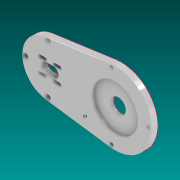
# Autodesk Inventor part: base bovenkant
Saved by Autodesk Inventor 2020.2 (Build 242310000, 310)
## iProperties
Created: 2020-05-15
Part Number: base bovenkant
Material: Aluminum 6061
Document SubType Name: Modeling
Designer: Svend
Density: 2.7 g/cm^3
Appearance: Aluminum - Polished
Author: Svend
Autodesk Inventor part; units mm, degrees
ref_plane "YZ Plane" through (0, 0, 0) normal (1, 0, 0) x (0, 1, 0)
ref_plane "XZ Plane" through (0, 0, 0) normal (0, 1, 0) x (-1, 0, 0)
ref_plane "XY Plane" through (0, 0, 0) normal (0, 0, 1) x (1, 0, 0)
sketch "Sketch1" plane through (0, 0, 0) normal (0, 0, 1) x (1, 0, 0)
  circle A0 centre (-11.3135, -11.3135) radius 2
  circle A1 centre (-11.3135, 11.3135) radius 2
  circle A2 centre (11.3135, 11.3135) radius 2
  circle A3 centre (11.3135, -11.3135) radius 2
  circle A4 centre (-15.3135, 11.3135) radius 2
  circle A5 centre (-7.3135, 11.3135) radius 2
  circle A6 centre (7.3135, 11.3135) radius 2
  circle A7 centre (15.3135, 11.3135) radius 2
  circle A8 centre (15.3135, -11.3135) radius 2
  circle A9 centre (7.3135, -11.3135) radius 2
  circle A10 centre (-7.3135, -11.3135) radius 2
  circle A11 centre (-15.3135, -11.3135) radius 2
  line L0 (-15.3135, 13.3135) -> (-7.3135, 13.3135)
  line L1 (-7.3135, 9.3135) -> (-15.3135, 9.3135)
  line L2 (-15.3135, -9.3135) -> (-7.3135, -9.3135)
  line L3 (-7.3135, -13.3135) -> (-15.3135, -13.3135)
  line L4 (7.3135, -9.3135) -> (15.3135, -9.3135)
  line L5 (15.3135, -13.3135) -> (7.3135, -13.3135)
  line L6 (15.3135, 9.3135) -> (7.3135, 9.3135)
  line L7 (15.3135, 13.3135) -> (7.3135, 13.3135)
  circle A12 centre (0, 0) radius 8.25
  circle A13 centre (5, 0) radius 8.25
  circle A14 centre (-5, 0) radius 8.25
  line L8 (-5, 8.25) -> (5, 8.25)
  line L9 (5, -8.25) -> (-5, -8.25)
  circle A15 centre (0, 0) radius 42.5
  circle A16 centre (100.143, 0) radius 56.4372
  line L10 (-5.9149, 42.0864) -> (92.2885, 55.888)
  line L11 (-5.9149, -42.0864) -> (92.2885, -55.888)
  line L12 (-13.25, 0) -> (13.25, 0)
  circle A17 centre (100.143, 0) radius 11.5
  arc A18 (-5.9149, 42.0864) -> (-5.9149, -42.0864) centre (0, 0) ccw
  arc A19 (92.2885, -55.888) -> (92.2885, 55.888) centre (100.143, 0) ccw
  line L13 (-42.5, 0) -> (156.5802, 0)
  line L14 (92.2885, 55.888) -> (-5.9149, 42.0864)
  line L15 (-5.9149, -42.0864) -> (92.2885, -55.888)
  line L16 (-3.1314, 22.281) -> (95.0719, 36.0826)
  arc A20 (95.0719, -36.0826) -> (95.0719, 36.0826) centre (100.143, 0) ccw
  line L17 (95.0719, -36.0826) -> (-3.1314, -22.281)
  arc A21 (-3.1314, 22.281) -> (-3.1314, -22.281) centre (0, 0) ccw
  point P0 (151.5802, 0)
  point P1 (95.0719, 51.23)
  point P2 (95.0719, -51.23)
  point P3 (-37.5, 0)
  point P4 (-3.1314, 37.4284)
  point P5 (-3.1314, -37.4284)
  dimension "d0" = 4
  dimension "d1" = 22.627
  dimension "d2" = 22.627
  dimension "d3" = 11.3135
  dimension "d4" = 11.3135
  dimension "d5" = 4
  dimension "d6" = 4
  dimension "d7" = 4
  dimension "d8" = 4
  dimension "d9" = 4
  dimension "d10" = 4
  dimension "d11" = 4
  dimension "d12" = 4
  dimension "d15" = 16.5
  dimension "d16" = 5
  dimension "d17" = 5
  dimension "d18" = 85
  dimension "d19" = 8
  dimension "d20" = 100.143
  dimension "d21" = 23
  dimension "d24" = 85
  dimension "d25" = 100.143
  dimension "d26" = 8
  dimension "d27" = 20
  dimension "d28" = 15
  dimension "d29" = 5
  dimension "d30" = 15
  dimension "d31" = 15
  dimension "d32" = 15
  dimension "d33" = 5
  constraints: 36 end point, 36 point on circle, 22 centre point, 15 horizontal alignment, 14 tangent, 13 equal radius, 11 point on line, 6 vertical alignment, 4 coincident, 4 parallel, 3 horizontal, 1 midpoint, 3 other
  measures "d0" diameter of A0
  measures "d1" distance of A1.centre A2.centre
  measures "d2" distance of A3.centre A2.centre
  measures "d3" horizontal distance of point (0, 0) A1.centre
  measures "d4" horizontal distance of point (0, 0) A1.centre
  measures "d5" distance of A2.centre A6.centre
  measures "d6" distance of A7.centre A2.centre
  measures "d7" distance of A3.centre A8.centre
  measures "d8" distance of A9.centre A3.centre
  measures "d9" distance of A0.centre A10.centre
  measures "d10" distance of A11.centre A0.centre
  measures "d11" distance of A1.centre A4.centre
  measures "d12" distance of A5.centre A1.centre
  measures "d15" diameter of A12
  measures "d16" distance of A14.centre A12.centre
  measures "d17" distance of A12.centre A13.centre
  measures "d18" diameter of A15
  measures "d19" angle of L12 L10
  measures "d20" distance of A16.centre point (0, 0)
  measures "d21" diameter of A17
  measures "d24" diameter of A18
  measures "d25" distance of A18.centre A19.centre
  measures "d26" angle of L13 L14
  measures "d27" distance between parallel lines of L14 L16
  measures "d28" distance from line of point (-3.131, -37.428) L17
  measures "d29" distance of L13.end point (151.58, 0)
  measures "d30" distance from line of L16 point (95.072, 51.23)
  measures "d31" distance from line of L16 point (-3.131, 37.428)
  measures "d32" distance from line of point (95.072, -51.23) L17
  measures "d33" distance of L13.start point (-37.5, 0)
extrude "Extrusion1" add sketch "Sketch1" along normal blind 10 contours L13 A15 L17 A21 A14 L9 A13 | A13 L8 A14 L13 A21 L16 A15 | L13 A16 L17 A15 | A15 L16 A16 L13 | L16 A21 L13 A15 | A15 L10 A16 L16 | L17 A16 L11 A15 | A15 L13 A21 L17 | L13 A17 A20 L17 A16 | A16 L16 A20 L13 A17 | A16 L13 A20 L16 | L17 A20 L13 A16
hole "Hole1" at (-3.1314, -37.4284, 0) at (95.0719, -51.23, 0) at (151.5802, 0, 0) at (95.0719, 51.23, 0) at (-3.1314, 37.4284, 0) at (-37.5, 0, 0) direction (0, 0, 1) diameter 5.2 depth 10 tip angle 118
chamfer "Chamfer1" distance 0.5 angle 45 28 edges at (-42.5, 0, 10) (43.1868, -48.9872, 10) (156.5802, 0, 10) (43.1868, 48.9872, 10) (-5.3135, 11.3135, 10) (-11.3135, 9.3135, 10) (-17.3135, 11.3135, 10) (-11.3135, 13.3135, 10) (-13.25, 0, 10) (0, 8.25, 10) (13.25, 0, 10) (0, -8.25, 10) (-11.3135, -9.3135, 10) (-5.3135, -11.3135, 10) (-11.3135, -13.3135, 10) (-17.3135, -11.3135, 10) (5.3135, 11.3135, 10) (11.3135, 13.3135, 10) (17.3135, 11.3135, 10) (11.3135, 9.3135, 10) (17.3135, -11.3135, 10) (11.3135, -13.3135, 10) (5.3135, -11.3135, 10) (11.3135, -9.3135, 10) (88.643, 0, 10) (95.0719, -53.83, 10) (151.5802, -2.6, 10) (95.0719, 48.63, 10)
chamfer "Chamfer3" distance 2 angle 45 3 edges at (-3.1314, 34.8284, 10) (-37.5, -2.6, 10) (-3.1314, -40.0284, 10)
sketch "Sketch2" plane through (0, 0, 10) normal (0, 0, 1) x (1, 0, 0)
  arc A0 (-41.9879, -1.0095) -> (-41.9879, 1.0095) centre (-37.5, 0) ccw projected
  circle A1 centre (95.0719, 51.23) radius 3.1 projected
  circle A2 centre (95.0719, -51.23) radius 3.1 projected
  arc A3 (15.3135, -13.8135) -> (15.3135, -8.8135) centre (15.3135, -11.3135) ccw projected
  line L0 (7.3135, -13.8135) -> (15.3135, -13.8135) projected
  arc A4 (7.3135, -8.8135) -> (7.3135, -13.8135) centre (7.3135, -11.3135) ccw projected
  line L1 (15.3135, -8.8135) -> (7.3135, -8.8135) projected
  line L2 (-7.3135, -8.8135) -> (-15.3135, -8.8135) projected
  arc A5 (-7.3135, -13.8135) -> (-7.3135, -8.8135) centre (-7.3135, -11.3135) ccw projected
  line L3 (-15.3135, -13.8135) -> (-7.3135, -13.8135) projected
  arc A6 (-15.3135, -8.8135) -> (-15.3135, -13.8135) centre (-15.3135, -11.3135) ccw projected
  arc A7 (-7.3135, 8.8135) -> (-7.3135, 13.8135) centre (-7.3135, 11.3135) ccw projected
  line L4 (-15.3135, 8.8135) -> (-7.3135, 8.8135) projected
  arc A8 (-15.3135, 13.8135) -> (-15.3135, 8.8135) centre (-15.3135, 11.3135) ccw projected
  line L5 (-7.3135, 13.8135) -> (-15.3135, 13.8135) projected
  arc A9 (-41.9879, -1.0095) -> (-5.8453, -41.5913) centre (0, 0) ccw projected
  line L6 (92.358, -55.3928) -> (-2.813, -42.0174) projected
  arc A10 (92.358, -55.3928) -> (92.358, 55.3928) centre (100.143, 0) ccw projected
  line L7 (-5.8453, 41.5913) -> (-4.7023, 41.7519) projected
  arc A11 (-5, 8.75) -> (-5, -8.75) centre (-5, 0) ccw projected
  line L8 (5, 8.75) -> (-5, 8.75) projected
  arc A12 (5, -8.75) -> (5, 8.75) centre (5, 0) ccw projected
  line L9 (-5, -8.75) -> (5, -8.75) projected
  arc A13 (7.3135, 13.8135) -> (7.3135, 8.8135) centre (7.3135, 11.3135) ccw projected
  line L10 (15.3135, 13.8135) -> (7.3135, 13.8135) projected
  arc A14 (15.3135, 8.8135) -> (15.3135, 13.8135) centre (15.3135, 11.3135) ccw projected
  line L11 (7.3135, 8.8135) -> (15.3135, 8.8135) projected
  circle A15 centre (100.143, 0) radius 12 projected
  circle A16 centre (151.5802, 0) radius 3.1 projected
  arc A17 (-4.7023, 41.7519) -> (-2.813, 42.0174) centre (-3.1314, 37.4284) ccw projected
  arc A18 (-2.813, -42.0174) -> (-4.7023, -41.7519) centre (-3.1314, -37.4284) ccw projected
  circle A19 centre (100.143, 0) radius 35.05
  line L12 (-2.813, 42.0174) -> (92.358, 55.3928) projected
  arc A20 (-5.8453, 41.5913) -> (-41.9879, 1.0095) centre (0, 0) ccw projected
  line L13 (-4.7023, -41.7519) -> (-5.8453, -41.5913) projected
  dimension "d50" = 70.1
  constraints: 1 centre point, 1 coincident
  measures "d50" diameter of A19
extrude "Extrusion2" cut sketch "Sketch2" against normal blind 5 contours A15 | A19
chamfer "Chamfer4" distance 1 angle 45 2 edges at (65.093, 0, 10) (88.643, 0, 5)
sketch "Sketch3" plane through (0, 0, 0) normal (0, 0, -1) x (-1, 0, 0)
  circle A0 centre (3.1314, 37.4284) radius 2.6 projected
  circle A1 centre (-151.5802, 0) radius 2.6 projected
  circle A2 centre (3.1314, -37.4284) radius 2.6 projected
  circle A3 centre (-95.0719, -51.23) radius 2.6 projected
  circle A4 centre (-95.0719, 51.23) radius 2.6 projected
  circle A5 centre (37.5, 0) radius 2.6 projected
  line L0 (5.9149, -42.0864) -> (-92.2885, -55.888) projected
  arc A6 (5.9149, -42.0864) -> (5.9149, 42.0864) centre (0, 0) ccw projected
  line L1 (-92.2885, 55.888) -> (5.9149, 42.0864) projected
  arc A7 (-92.2885, 55.888) -> (-92.2885, -55.888) centre (-100.143, 0) ccw projected
  circle A8 centre (-100.143, 0) radius 11.5 projected
  line L2 (7.3135, 9.3135) -> (15.3135, 9.3135) projected
  arc A9 (7.3135, 13.3135) -> (7.3135, 9.3135) centre (7.3135, 11.3135) ccw projected
  line L3 (15.3135, 13.3135) -> (7.3135, 13.3135) projected
  arc A10 (15.3135, 9.3135) -> (15.3135, 13.3135) centre (15.3135, 11.3135) ccw projected
  line L4 (7.3135, -13.3135) -> (15.3135, -13.3135) projected
  arc A11 (7.3135, -9.3135) -> (7.3135, -13.3135) centre (7.3135, -11.3135) ccw projected
  line L5 (15.3135, -9.3135) -> (7.3135, -9.3135) projected
  arc A12 (15.3135, -13.3135) -> (15.3135, -9.3135) centre (15.3135, -11.3135) ccw projected
  line L6 (-15.3135, -13.3135) -> (-7.3135, -13.3135) projected
  arc A13 (-15.3135, -9.3135) -> (-15.3135, -13.3135) centre (-15.3135, -11.3135) ccw projected
  line L7 (-7.3135, -9.3135) -> (-15.3135, -9.3135) projected
  arc A14 (-7.3135, -13.3135) -> (-7.3135, -9.3135) centre (-7.3135, -11.3135) ccw projected
  line L8 (-7.3135, 13.3135) -> (-15.3135, 13.3135) projected
  arc A15 (-7.3135, 9.3135) -> (-7.3135, 13.3135) centre (-7.3135, 11.3135) ccw projected
  line L9 (-15.3135, 9.3135) -> (-7.3135, 9.3135) projected
  arc A16 (-15.3135, 13.3135) -> (-15.3135, 9.3135) centre (-15.3135, 11.3135) ccw projected
  line L10 (-5, -8.25) -> (5, -8.25) projected
  arc A17 (-5, 8.25) -> (-5, -8.25) centre (-5, 0) ccw projected
  line L11 (5, 8.25) -> (-5, 8.25) projected
  arc A18 (5, -8.25) -> (5, 8.25) centre (5, 0) ccw projected
  line L12 (-93.6802, -45.9853) -> (4.5231, -32.1837)
  arc A19 (4.5231, -32.1837) -> (4.5231, 32.1837) centre (0, 0) ccw
  line L13 (4.5231, 32.1837) -> (-93.6802, 45.9853)
  arc A20 (-93.6802, 45.9853) -> (-93.6802, -45.9853) centre (-100.143, 0) ccw
  dimension "d56" = 10
  constraints: 4 end point, 4 point on circle, 2 centre point, 3 other
  measures "d56" distance between parallel lines of L0 L12
equation "\"d2\" = d1"
equation "\"d3\" = 0.5 * d2"
equation "\"d4\" = 0.5 * d1"
equation "\"d5\" = d0"
equation "\"d6\" = d5"
equation "\"d7\" = d6"
equation "\"d8\" = d7"
equation "\"d9\" = d5"
equation "\"d10\" = d9"
equation "\"d11\" = d10"
equation "\"d12\" = d11"
equation "\"d17\" = d16"
equation "\"d32\" = d30"
equation "\"d35\" = d32"
body "Solid1"
